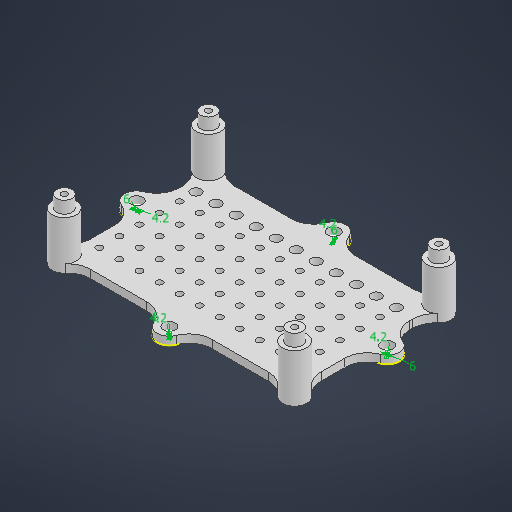
# Autodesk Inventor part: Bottom_Tip_Matrix
Saved by Autodesk Inventor 2025.1 (Build 291241000, 241)
## iProperties
Created: 2025-02-14
Part Number: Bottom_Tip_Matrix
Material: Generic
Document SubType Name: Modeling
Designer: m_kni
Density: 1 g/cm^3
Appearance: Default
Author: m_kni
## iProperties of the stored document Bottom_Tip_Matrix_3DPrint.ipt
Created: 2025-02-16
Part Number: Bottom_Tip_Matrix_3DPrint
Material: Generic
Document SubType Name: Modeling
Designer: m_kni
Density: 1 g/cm^3
Appearance: Default
Author: m_kni
Autodesk Inventor part; units mm, degrees
ref_plane "YZ Plane" through (0, 0, 0) normal (1, 0, 0) x (0, 1, 0)
ref_plane "XZ Plane" through (0, 0, 0) normal (0, 1, 0) x (-1, 0, 0)
ref_plane "XY Plane" through (0, 0, 0) normal (0, 0, 1) x (1, 0, 0)
sketch "Sketch1" plane through (0, 0, 0) normal (0, 1, 0) x (-1, 0, 0)
  line L0 (63.6935, -29.7828) -> (-51.3065, -29.7828)
  line L1 (-51.3065, -29.7828) -> (-51.3065, 42.2172)
  line L2 (-51.3065, 42.2172) -> (63.6935, 42.2172)
  line L3 (63.6935, -29.7828) -> (-51.3065, 42.2172) construction
  line L4 (-51.3065, -29.7828) -> (63.6935, 42.2172) construction
  circle A0 centre (-42.3065, 30.6406) radius 1.6
  circle A1 centre (-42.3065, 20.6406) radius 1.6
  circle A2 centre (-42.3065, 10.6406) radius 1.6
  circle A3 centre (-42.3065, 0.6406) radius 1.6
  circle A4 centre (-42.3065, -9.3594) radius 1.6
  circle A5 centre (-32.3065, 30.6406) radius 1.6
  circle A6 centre (-32.3065, 20.6406) radius 1.6
  circle A7 centre (-32.3065, 10.6406) radius 1.6
  circle A8 centre (-32.3065, 0.6406) radius 1.6
  circle A9 centre (-32.3065, -9.3594) radius 1.6
  circle A10 centre (-22.3065, 30.6406) radius 1.6
  circle A11 centre (-22.3065, 20.6406) radius 1.6
  circle A12 centre (-22.3065, 10.6406) radius 1.6
  circle A13 centre (-22.3065, 0.6406) radius 1.6
  circle A14 centre (-22.3065, -9.3594) radius 1.6
  circle A15 centre (-12.3065, 30.6406) radius 1.6
  circle A16 centre (-12.3065, 20.6406) radius 1.6
  circle A17 centre (-12.3065, 10.6406) radius 1.6
  circle A18 centre (-12.3065, 0.6406) radius 1.6
  circle A19 centre (-12.3065, -9.3594) radius 1.6
  circle A20 centre (-2.3065, 30.6406) radius 1.6
  circle A21 centre (-2.3065, 20.6406) radius 1.6
  circle A22 centre (-2.3065, 10.6406) radius 1.6
  circle A23 centre (-2.3065, 0.6406) radius 1.6
  circle A24 centre (-2.3065, -9.3594) radius 1.6
  circle A25 centre (7.6935, 30.6406) radius 1.6
  circle A26 centre (7.6935, 20.6406) radius 1.6
  circle A27 centre (7.6935, 10.6406) radius 1.6
  circle A28 centre (7.6935, 0.6406) radius 1.6
  circle A29 centre (7.6935, -9.3594) radius 1.6
  circle A30 centre (17.6935, 30.6406) radius 1.6
  circle A31 centre (17.6935, 20.6406) radius 1.6
  circle A32 centre (17.6935, 10.6406) radius 1.6
  circle A33 centre (17.6935, 0.6406) radius 1.6
  circle A34 centre (17.6935, -9.3594) radius 1.6
  circle A35 centre (27.6935, 30.6406) radius 1.6
  circle A36 centre (27.6935, 20.6406) radius 1.6
  circle A37 centre (27.6935, 10.6406) radius 1.6
  circle A38 centre (27.6935, 0.6406) radius 1.6
  circle A39 centre (27.6935, -9.3594) radius 1.6
  circle A40 centre (37.6935, 30.6406) radius 1.6
  circle A41 centre (37.6935, 20.6406) radius 1.6
  circle A42 centre (37.6935, 10.6406) radius 1.6
  circle A43 centre (37.6935, 0.6406) radius 1.6
  circle A44 centre (37.6935, -9.3594) radius 1.6
  circle A45 centre (47.6935, 30.6406) radius 1.6
  circle A46 centre (47.6935, 20.6406) radius 1.6
  circle A47 centre (47.6935, 10.6406) radius 1.6
  circle A48 centre (47.6935, 0.6406) radius 1.6
  circle A49 centre (47.6935, -9.3594) radius 1.6
  circle A50 centre (57.6935, 30.6406) radius 1.6
  circle A51 centre (57.6935, 20.6406) radius 1.6
  circle A52 centre (57.6935, 10.6406) radius 1.6
  circle A53 centre (57.6935, 0.6406) radius 1.6
  circle A54 centre (57.6935, -9.3594) radius 1.6
  line L5 (-51.3065, 42.2172) -> (63.6935, 42.2172)
  line L6 (63.6935, 42.2172) -> (63.6935, -29.7828)
  line L7 (63.6935, -29.7828) -> (-51.3065, -29.7828)
  line L8 (-51.3065, -29.7828) -> (-51.3065, 42.2172)
  circle A55 centre (-51.3065, 42.2172) radius 6
  circle A56 centre (-51.3065, -29.7828) radius 6
  circle A57 centre (63.6935, 42.2172) radius 6
  circle A58 centre (63.6935, -29.7828) radius 6
  circle A59 centre (57.6935, -17.5594) radius 2.5
  line L9 (57.6935, -9.3594) -> (57.6935, -17.5594) construction
  circle A60 centre (47.6935, -17.5594) radius 2.5
  circle A61 centre (37.6935, -17.5594) radius 2.5
  circle A62 centre (27.6935, -17.5594) radius 2.5
  circle A63 centre (17.6935, -17.5594) radius 2.5
  circle A64 centre (7.6935, -17.5594) radius 2.5
  circle A65 centre (-2.3065, -17.5594) radius 2.5
  circle A66 centre (-12.3065, -17.5594) radius 2.5
  circle A67 centre (-22.3065, -17.5594) radius 2.5
  circle A68 centre (-32.3065, -17.5594) radius 2.5
  circle A69 centre (-42.3065, -17.5594) radius 2.5
  point P0 (0, 0)
  point P1 (6.1935, 6.2172)
  point P2 (60.4545, 30.6406)
  point P3 (-45.5455, -35.3594)
  point P4 (63.6935, -23.7828)
  point P5 (63.6935, 36.2172)
  point P6 (57.6935, 42.2172)
  point P7 (-45.3065, 42.2172)
  point P8 (-51.3065, 36.2172)
  point P9 (-51.3065, -23.7828)
  point P10 (-45.3065, -29.7828)
  point P11 (57.6935, -29.7828)
  dimension "d4" = 115
  dimension "d5" = 72
  dimension "d6" = 3.2
  dimension "d9" = 10
  dimension "d10" = 10
  dimension "d13" = 12
  dimension "d14" = 12
  dimension "d15" = 12
  dimension "d16" = 12
  dimension "d58" = 6
  dimension "d59" = 8.2
  dimension "d60" = 5
  dimension "d63" = 10
  constraints: 70 centre point, 20 end point, 5 coincident, 4 horizontal, 3 parallel, 2 midpoint, 2 perpendicular, 2 vertical, 1 point on line, 128 other
  measures "d4" distance of L1.end L4.end
  measures "d5" distance of L1.start L1.end
  measures "d6" diameter of A0
  measures "d9" distance of A0.centre A1.centre
  measures "d10" distance of A0.centre A5.centre
  measures "d13" diameter of A55
  measures "d14" diameter of A56
  measures "d15" diameter of A57
  measures "d16" diameter of A58
  measures "d58" distance from line of L6 A50.centre
  measures "d59" distance of L9.start L9.end
  measures "d60" diameter of A59
  measures "d63" distance of L9.end A60.centre
extrude "Extrusion1" add sketch "Sketch1" along normal blind 4
sketch "Sketch2" plane through (0, 4, 0) normal (0, 1, 0) x (1, 0, 0)
  arc A0 (45.3065, -42.2172) -> (51.3065, -36.2172) centre (51.3065, -42.2172) ccw projected
  arc A1 (-63.6935, -36.2172) -> (-57.6935, -42.2172) centre (-63.6935, -42.2172) ccw projected
  arc A2 (-57.6935, 29.7828) -> (-63.6935, 23.7828) centre (-63.6935, 29.7828) ccw projected
  arc A3 (51.3065, 23.7828) -> (45.3065, 29.7828) centre (51.3065, 29.7828) ccw projected
  circle A4 centre (-63.6935, -42.2172) radius 6
  circle A5 centre (-63.6935, 29.7828) radius 6
  circle A6 centre (51.3065, -42.2172) radius 6
  circle A7 centre (51.3065, 29.7828) radius 6
  point P0 (0, 0)
  point P1 (51.3065, 23.7828)
  point P2 (45.3065, -42.2172)
  point P3 (-57.6935, 29.7828)
  constraints: 4 coincident, 3 centre point, 3 concentric, 3 other
extrude "Extrusion2" add sketch "Sketch2" along normal blind 20
sketch "Sketch3" plane through (51.3065, 24, 42.2172) normal (0, 1, 0) x (1, 0, 0)
  circle A0 centre (0, 0) radius 3.85
  arc A1 (0, 66) -> (-6, 72) centre (0, 72) ccw projected
  circle A2 centre (0, 72) radius 3.85
  arc A3 (-115, 6) -> (-109, 0) centre (-115, 0) ccw projected
  circle A4 centre (-115, 0) radius 3.85
  circle A5 centre (-115, 72) radius 3.85
  circle A6 centre (-115, 72) radius 6 projected
  point P0 (-51.3065, 42.2172)
  dimension "d21" = 7.7
  dimension "d22" = 7.7
  dimension "d23" = 7.7
  dimension "d24" = 7.7
  constraints: 4 centre point, 3 coincident
  measures "d21" diameter of A0
  measures "d22" diameter of A2
  measures "d23" diameter of A4
  measures "d24" diameter of A5
extrude "Extrusion3" add sketch "Sketch3" along normal blind 6 contours A0 | A2 | A4 | A5
sketch "Sketch4" plane through (-63.6935, 30, 42.2172) normal (0, 1, 0) x (1, 0, 0)
  circle A0 centre (0, 0) radius 3.85 projected
  circle A1 centre (0, 72) radius 3.85 projected
  circle A2 centre (115, 0) radius 3.85 projected
  circle A3 centre (115, 72) radius 3.85 projected
  circle A4 centre (0, 0) radius 1.5
  circle A5 centre (115, 0) radius 1.5
  circle A6 centre (0, 72) radius 1.5
  circle A7 centre (115, 72) radius 1.5
  point P0 (63.6935, 42.2172)
  dimension "d27" = 3
  dimension "d28" = 3
  dimension "d29" = 3
  dimension "d30" = 3
  constraints: 4 centre point, 4 coincident
  measures "d27" diameter of A4
  measures "d28" diameter of A5
  measures "d29" diameter of A6
  measures "d30" diameter of A7
extrude "Extrusion4" cut sketch "Sketch4" against normal blind 8 contours A4 | A5 | A6 | A7
sketch "Sketch5" plane through (0, 4, 0) normal (0, 1, 0) x (1, 0, 0)
  line L0 (-57.6935, -42.2172) -> (45.3065, -42.2172) projected
  line L1 (-6.1935, -42.2172) -> (-6.1935, -47.2172)
  circle A0 centre (-6.1935, -47.2172) radius 6
  line L2 (45.3065, 29.7828) -> (-57.6935, 29.7828) projected
  line L3 (-63.6935, 23.7828) -> (-63.6935, -36.2172) projected
  line L4 (51.3065, -36.2172) -> (51.3065, 23.7828) projected
  circle A1 centre (56.3065, -1.0083) radius 6
  circle A2 centre (-6.1935, 34.7828) radius 6
  circle A3 centre (-68.6935, -1.0083) radius 6
  line L5 (56.3065, -7.0083) -> (51.3065, -7.0083)
  line L6 (56.3065, 4.9917) -> (51.3065, 4.9917)
  line L7 (-68.6935, 4.9917) -> (-63.6935, 4.9917)
  line L8 (-68.6935, -7.0083) -> (-63.6935, -7.0083)
  line L9 (-12.1935, -47.2172) -> (-12.1935, -42.2172)
  line L10 (-0.1935, -47.2172) -> (-0.1935, -42.2172)
  line L11 (-12.1935, 34.7828) -> (-12.1935, 29.7828)
  line L12 (-0.1935, 34.7828) -> (-0.1935, 29.7828)
  line L13 (-12.1935, -42.2172) -> (-12.7108, -42.2172)
  circle A4 centre (42.3065, -10.6406) radius 1.6 projected
  circle A5 centre (42.3065, -0.6406) radius 1.6 projected
  circle A6 centre (32.3065, -10.6406) radius 1.6 projected
  circle A7 centre (32.3065, -30.6406) radius 1.6 projected
  circle A8 centre (32.3065, -10.6406) radius 1.6 projected
  circle A9 centre (32.3065, 9.3594) radius 1.6 projected
  circle A10 centre (32.3065, 9.3594) radius 1.6 projected
  circle A11 centre (32.3065, 9.3594) radius 1.6 projected
  circle A12 centre (32.3065, 9.3594) radius 1.6 projected
  circle A13 centre (32.3065, 19.3594) radius 1.6 projected
  circle A14 centre (42.3065, 9.3594) radius 1.6 projected
  arc A15 (45.3065, -42.2172) -> (51.3065, -36.2172) centre (51.3065, -42.2172) ccw projected
  arc A16 (51.3065, -36.2172) -> (45.3065, -42.2172) centre (51.3065, -42.2172) ccw projected
  arc A17 (45.3065, 29.7828) -> (51.3065, 23.7828) centre (51.3065, 29.7828) ccw projected
  circle A18 centre (2.3065, 19.3594) radius 1.6 projected
  circle A19 centre (2.3065, 19.3594) radius 1.6 projected
  circle A20 centre (51.3065, 29.7828) radius 3.85 projected
  circle A21 centre (51.3065, 29.7828) radius 1.5 projected
  circle A22 centre (51.3065, 29.7828) radius 1.5 projected
  circle A23 centre (51.3065, 29.7828) radius 1.5 projected
  circle A24 centre (51.3065, 29.7828) radius 3.85 projected
  circle A25 centre (51.3065, 29.7828) radius 1.5 projected
  circle A26 centre (51.3065, 29.7828) radius 1.5 projected
  circle A27 centre (51.3065, 29.7828) radius 1.5 projected
  circle A28 centre (2.3065, 29.3594) radius 1.6 projected
  circle A29 centre (2.3065, 29.3594) radius 1.6 projected
  circle A30 centre (2.3065, 29.3594) radius 1.6 projected
  circle A31 centre (2.3065, 29.3594) radius 1.6 projected
  circle A32 centre (12.3065, 29.3594) radius 1.6 projected
  circle A33 centre (12.3065, 29.3594) radius 1.6 projected
  circle A34 centre (12.3065, 9.3594) radius 1.6 projected
  circle A35 centre (12.3065, 9.3594) radius 1.6 projected
  circle A36 centre (12.3065, 9.3594) radius 1.6 projected
  circle A37 centre (12.3065, 9.3594) radius 1.6 projected
  circle A38 centre (12.3065, 19.3594) radius 1.6 projected
  circle A39 centre (12.3065, 19.3594) radius 1.6 projected
  circle A40 centre (12.3065, 19.3594) radius 1.6 projected
  circle A41 centre (12.3065, 29.3594) radius 1.6 projected
  circle A42 centre (12.3065, 29.3594) radius 1.6 projected
  circle A43 centre (2.3065, 9.3594) radius 1.6 projected
  circle A44 centre (2.3065, 9.3594) radius 1.6 projected
  circle A45 centre (2.3065, 19.3594) radius 1.6 projected
  circle A46 centre (2.3065, 19.3594) radius 1.6 projected
  circle A47 centre (2.3065, 9.3594) radius 1.6 projected
  circle A48 centre (12.3065, 19.3594) radius 1.6 projected
  circle A49 centre (22.3065, 29.3594) radius 1.6 projected
  arc A50 (51.3065, 23.7828) -> (45.3065, 29.7828) centre (51.3065, 29.7828) ccw projected
  circle A51 centre (22.3065, 9.3594) radius 1.6 projected
  circle A52 centre (-7.6935, -0.6406) radius 1.6 projected
  circle A53 centre (-7.6935, -0.6406) radius 1.6 projected
  circle A54 centre (-7.6935, -10.6406) radius 1.6 projected
  circle A55 centre (-17.6935, -10.6406) radius 1.6 projected
  circle A56 centre (-17.6935, -10.6406) radius 1.6 projected
  circle A57 centre (51.3065, -42.2172) radius 1.5 projected
  circle A58 centre (42.3065, 9.3594) radius 1.6 projected
  circle A59 centre (42.3065, 9.3594) radius 1.6 projected
  circle A60 centre (51.3065, -42.2172) radius 3.85 projected
  circle A61 centre (42.3065, 19.3594) radius 1.6 projected
  circle A62 centre (42.3065, 19.3594) radius 1.6 projected
  circle A63 centre (-7.6935, 9.3594) radius 1.6 projected
  circle A64 centre (-17.6935, 9.3594) radius 1.6 projected
  circle A65 centre (-17.6935, 9.3594) radius 1.6 projected
  circle A66 centre (-7.6935, 9.3594) radius 1.6 projected
  circle A67 centre (-7.6935, -20.6406) radius 1.6 projected
  circle A68 centre (-7.6935, -20.6406) radius 1.6 projected
  circle A69 centre (12.3065, -20.6406) radius 1.6 projected
  circle A70 centre (2.3065, -30.6406) radius 1.6 projected
  circle A71 centre (-7.6935, -30.6406) radius 1.6 projected
  circle A72 centre (-7.6935, -30.6406) radius 1.6 projected
  circle A73 centre (-17.6935, -20.6406) radius 1.6 projected
  circle A74 centre (-17.6935, -20.6406) radius 1.6 projected
  circle A75 centre (12.3065, -20.6406) radius 1.6 projected
  circle A76 centre (2.3065, -0.6406) radius 1.6 projected
  circle A77 centre (-17.6935, -30.6406) radius 1.6 projected
  circle A78 centre (-17.6935, -30.6406) radius 1.6 projected
  circle A79 centre (2.3065, -0.6406) radius 1.6 projected
  circle A80 centre (-7.6935, 19.3594) radius 1.6 projected
  circle A81 centre (-7.6935, 19.3594) radius 1.6 projected
  circle A82 centre (-7.6935, 29.3594) radius 1.6 projected
  circle A83 centre (-7.6935, 29.3594) radius 1.6 projected
  circle A84 centre (-17.6935, 19.3594) radius 1.6 projected
  circle A85 centre (-17.6935, 19.3594) radius 1.6 projected
  circle A86 centre (-7.6935, 19.3594) radius 1.6 projected
  circle A87 centre (-7.6935, 19.3594) radius 1.6 projected
  circle A88 centre (-7.6935, 29.3594) radius 1.6 projected
  circle A89 centre (-7.6935, 29.3594) radius 1.6 projected
  circle A90 centre (-17.6935, -0.6406) radius 1.6 projected
  circle A91 centre (-17.6935, -0.6406) radius 1.6 projected
  circle A92 centre (51.3065, -42.2172) radius 3.85 projected
  circle A93 centre (51.3065, -42.2172) radius 1.5 projected
  circle A94 centre (51.3065, -42.2172) radius 1.5 projected
  circle A95 centre (51.3065, -42.2172) radius 3.85 projected
  circle A96 centre (51.3065, -42.2172) radius 1.5 projected
  circle A97 centre (51.3065, -42.2172) radius 1.5 projected
  circle A98 centre (32.3065, -30.6406) radius 1.6 projected
  circle A99 centre (32.3065, -30.6406) radius 1.6 projected
  circle A100 centre (32.3065, -0.6406) radius 1.6 projected
  circle A101 centre (32.3065, -0.6406) radius 1.6 projected
  circle A102 centre (32.3065, -10.6406) radius 1.6 projected
  circle A103 centre (32.3065, -10.6406) radius 1.6 projected
  circle A104 centre (32.3065, -20.6406) radius 1.6 projected
  circle A105 centre (32.3065, -20.6406) radius 1.6 projected
  circle A106 centre (42.3065, -20.6406) radius 1.6 projected
  circle A107 centre (42.3065, -20.6406) radius 1.6 projected
  circle A108 centre (42.3065, -10.6406) radius 1.6 projected
  circle A109 centre (42.3065, -10.6406) radius 1.6 projected
  circle A110 centre (42.3065, -30.6406) radius 1.6 projected
  circle A111 centre (42.3065, -30.6406) radius 1.6 projected
  circle A112 centre (51.3065, -42.2172) radius 3.85 projected
  circle A113 centre (51.3065, -42.2172) radius 3.85 projected
  circle A114 centre (51.3065, -42.2172) radius 6 projected
  circle A115 centre (51.3065, -42.2172) radius 6 projected
  arc A116 (45.3065, -42.2172) -> (51.3065, -36.2172) centre (51.3065, -42.2172) ccw projected
  arc A117 (51.3065, -36.2172) -> (45.3065, -42.2172) centre (51.3065, -42.2172) ccw projected
  circle A118 centre (51.3065, -42.2172) radius 3.85 projected
  circle A119 centre (51.3065, -42.2172) radius 6 projected
  line L14 (51.3065, -36.2172) -> (51.3065, 23.7828) projected
  line L15 (51.3065, -36.2172) -> (51.3065, 23.7828) projected
  circle A120 centre (42.3065, -0.6406) radius 1.6 projected
  circle A121 centre (42.3065, -0.6406) radius 1.6 projected
  circle A122 centre (-27.6935, 19.3594) radius 1.6 projected
  circle A123 centre (-27.6935, 29.3594) radius 1.6 projected
  circle A124 centre (-27.6935, 29.3594) radius 1.6 projected
  circle A125 centre (-27.6935, 19.3594) radius 1.6 projected
  circle A126 centre (-47.6935, -20.6406) radius 1.6 projected
  circle A127 centre (-47.6935, -20.6406) radius 1.6 projected
  circle A128 centre (-47.6935, -30.6406) radius 1.6 projected
  circle A129 centre (-47.6935, -30.6406) radius 1.6 projected
  circle A130 centre (-37.6935, -20.6406) radius 1.6 projected
  circle A131 centre (-37.6935, -20.6406) radius 1.6 projected
  circle A132 centre (-27.6935, 9.3594) radius 1.6 projected
  circle A133 centre (-27.6935, 9.3594) radius 1.6 projected
  circle A134 centre (-37.6935, -0.6406) radius 1.6 projected
  circle A135 centre (-37.6935, -0.6406) radius 1.6 projected
  circle A136 centre (-27.6935, -30.6406) radius 1.6 projected
  circle A137 centre (-27.6935, -30.6406) radius 1.6 projected
  circle A138 centre (-27.6935, -10.6406) radius 1.6 projected
  circle A139 centre (-27.6935, -10.6406) radius 1.6 projected
  circle A140 centre (-27.6935, -0.6406) radius 1.6 projected
  circle A141 centre (-27.6935, -0.6406) radius 1.6 projected
  circle A142 centre (-37.6935, 9.3594) radius 1.6 projected
  circle A143 centre (-27.6935, -20.6406) radius 1.6 projected
  circle A144 centre (-27.6935, -20.6406) radius 1.6 projected
  circle A145 centre (-37.6935, -10.6406) radius 1.6 projected
  circle A146 centre (-37.6935, -10.6406) radius 1.6 projected
  circle A147 centre (-47.6935, -10.6406) radius 1.6 projected
  circle A148 centre (-37.6935, -30.6406) radius 1.6 projected
  circle A149 centre (-37.6935, -30.6406) radius 1.6 projected
  circle A150 centre (-37.6935, 9.3594) radius 1.6 projected
  circle A151 centre (-47.6935, -0.6406) radius 1.6 projected
  circle A152 centre (-47.6935, -0.6406) radius 1.6 projected
  circle A153 centre (-57.6935, 19.3594) radius 1.6 projected
  circle A154 centre (-57.6935, 19.3594) radius 1.6 projected
  circle A155 centre (-57.6935, 9.3594) radius 1.6 projected
  circle A156 centre (-57.6935, 9.3594) radius 1.6 projected
  circle A157 centre (-47.6935, 19.3594) radius 1.6 projected
  circle A158 centre (-47.6935, 19.3594) radius 1.6 projected
  circle A159 centre (-57.6935, -10.6406) radius 1.6 projected
  circle A160 centre (-37.6935, 19.3594) radius 1.6 projected
  circle A161 centre (-37.6935, 29.3594) radius 1.6 projected
  circle A162 centre (-37.6935, 29.3594) radius 1.6 projected
  circle A163 centre (-57.6935, -10.6406) radius 1.6 projected
  circle A164 centre (-37.6935, 19.3594) radius 1.6 projected
  circle A165 centre (-63.6935, -42.2172) radius 1.5 projected
  circle A166 centre (-63.6935, -42.2172) radius 1.5 projected
  circle A167 centre (-63.6935, -42.2172) radius 1.5 projected
  circle A168 centre (-63.6935, -42.2172) radius 1.5 projected
  circle A169 centre (-63.6935, -42.2172) radius 1.5 projected
  arc A170 (-57.6935, -42.2172) -> (-63.6935, -36.2172) centre (-63.6935, -42.2172) ccw projected
  arc A171 (-63.6935, -36.2172) -> (-57.6935, -42.2172) centre (-63.6935, -42.2172) ccw projected
  line L16 (-63.6935, 23.7828) -> (-63.6935, -36.2172) projected
  arc A172 (-63.6935, 23.7828) -> (-57.6935, 29.7828) centre (-63.6935, 29.7828) ccw projected
  arc A173 (-57.6935, 29.7828) -> (-63.6935, 23.7828) centre (-63.6935, 29.7828) ccw projected
  circle A174 centre (-63.6935, 29.7828) radius 3.85 projected
  circle A175 centre (-63.6935, 29.7828) radius 1.5 projected
  circle A176 centre (-63.6935, 29.7828) radius 1.5 projected
  circle A177 centre (-63.6935, 29.7828) radius 1.5 projected
  circle A178 centre (-63.6935, 29.7828) radius 3.85 projected
  circle A179 centre (-63.6935, 29.7828) radius 1.5 projected
  circle A180 centre (-63.6935, 29.7828) radius 1.5 projected
  circle A181 centre (-63.6935, 29.7828) radius 6 projected
  arc A182 (-57.6935, 29.7828) -> (-63.6935, 23.7828) centre (-63.6935, 29.7828) ccw projected
  arc A183 (-63.6935, 23.7828) -> (-57.6935, 29.7828) centre (-63.6935, 29.7828) ccw projected
  circle A184 centre (-57.6935, 19.3594) radius 1.6 projected
  circle A185 centre (-57.6935, 19.3594) radius 1.6 projected
  circle A186 centre (-57.6935, 9.3594) radius 1.6 projected
  circle A187 centre (-57.6935, 9.3594) radius 1.6 projected
  circle A188 centre (-47.6935, 19.3594) radius 1.6 projected
  circle A189 centre (-47.6935, 19.3594) radius 1.6 projected
  circle A190 centre (-17.6935, 9.3594) radius 1.6 projected
  circle A191 centre (-17.6935, 9.3594) radius 1.6 projected
  circle A192 centre (-37.6935, 9.3594) radius 1.6 projected
  circle A193 centre (-37.6935, 9.3594) radius 1.6 projected
  circle A194 centre (-47.6935, 9.3594) radius 1.6 projected
  circle A195 centre (-47.6935, 9.3594) radius 1.6 projected
  circle A196 centre (-37.6935, 19.3594) radius 1.6 projected
  circle A197 centre (-37.6935, 19.3594) radius 1.6 projected
  circle A198 centre (-63.6935, 29.7828) radius 3.85 projected
  circle A199 centre (-63.6935, 29.7828) radius 3.85 projected
  circle A200 centre (-63.6935, 29.7828) radius 3.85 projected
  circle A201 centre (-63.6935, 29.7828) radius 6 projected
  circle A202 centre (-57.6935, 29.3594) radius 1.6 projected
  circle A203 centre (-57.6935, 29.3594) radius 1.6 projected
  circle A204 centre (-27.6935, 19.3594) radius 1.6 projected
  circle A205 centre (-27.6935, 19.3594) radius 1.6 projected
  circle A206 centre (-47.6935, 29.3594) radius 1.6 projected
  circle A207 centre (-47.6935, 29.3594) radius 1.6 projected
  circle A208 centre (-37.6935, 29.3594) radius 1.6 projected
  circle A209 centre (-37.6935, 29.3594) radius 1.6 projected
  circle A210 centre (-17.6935, 19.3594) radius 1.6 projected
  circle A211 centre (-17.6935, 19.3594) radius 1.6 projected
  circle A212 centre (-27.6935, 29.3594) radius 1.6 projected
  circle A213 centre (-27.6935, 29.3594) radius 1.6 projected
  circle A214 centre (-17.6935, 29.3594) radius 1.6 projected
  circle A215 centre (-17.6935, 29.3594) radius 1.6 projected
  circle A216 centre (-27.6935, 9.3594) radius 1.6 projected
  circle A217 centre (-27.6935, 9.3594) radius 1.6 projected
  circle A218 centre (-63.6935, -42.2172) radius 3.85 projected
  circle A219 centre (-63.6935, -42.2172) radius 1.5 projected
  circle A220 centre (-63.6935, -42.2172) radius 3.85 projected
  circle A221 centre (-63.6935, -42.2172) radius 3.85 projected
  circle A222 centre (-63.6935, -42.2172) radius 6 projected
  arc A223 (-63.6935, -36.2172) -> (-57.6935, -42.2172) centre (-63.6935, -42.2172) ccw projected
  arc A224 (-57.6935, -42.2172) -> (-63.6935, -36.2172) centre (-63.6935, -42.2172) ccw projected
  line L17 (-63.6935, 23.7828) -> (-63.6935, -36.2172) projected
  line L18 (-63.6935, 23.7828) -> (-63.6935, -36.2172) projected
  circle A225 centre (-47.6935, -0.6406) radius 1.6 projected
  circle A226 centre (-47.6935, -0.6406) radius 1.6 projected
  circle A227 centre (-57.6935, -10.6406) radius 1.6 projected
  circle A228 centre (-57.6935, -10.6406) radius 1.6 projected
  circle A229 centre (-47.6935, -20.6406) radius 1.6 projected
  circle A230 centre (-47.6935, -20.6406) radius 1.6 projected
  circle A231 centre (-47.6935, -30.6406) radius 1.6 projected
  circle A232 centre (-47.6935, -30.6406) radius 1.6 projected
  circle A233 centre (-37.6935, -20.6406) radius 1.6 projected
  circle A234 centre (-37.6935, -20.6406) radius 1.6 projected
  circle A235 centre (-37.6935, -0.6406) radius 1.6 projected
  circle A236 centre (-37.6935, -0.6406) radius 1.6 projected
  circle A237 centre (-17.6935, -0.6406) radius 1.6 projected
  circle A238 centre (-17.6935, -0.6406) radius 1.6 projected
  circle A239 centre (-27.6935, -0.6406) radius 1.6 projected
  circle A240 centre (-27.6935, -0.6406) radius 1.6 projected
  circle A241 centre (-57.6935, -0.6406) radius 1.6 projected
  circle A242 centre (-57.6935, -0.6406) radius 1.6 projected
  circle A243 centre (-27.6935, -10.6406) radius 1.6 projected
  circle A244 centre (-27.6935, -10.6406) radius 1.6 projected
  circle A245 centre (-17.6935, -10.6406) radius 1.6 projected
  circle A246 centre (-17.6935, -10.6406) radius 1.6 projected
  circle A247 centre (-47.6935, -10.6406) radius 1.6 projected
  circle A248 centre (-47.6935, -10.6406) radius 1.6 projected
  circle A249 centre (-17.6935, -20.6406) radius 1.6 projected
  circle A250 centre (-17.6935, -20.6406) radius 1.6 projected
  circle A251 centre (-27.6935, -20.6406) radius 1.6 projected
  circle A252 centre (-27.6935, -20.6406) radius 1.6 projected
  circle A253 centre (-17.6935, -30.6406) radius 1.6 projected
  circle A254 centre (-17.6935, -30.6406) radius 1.6 projected
  circle A255 centre (-27.6935, -30.6406) radius 1.6 projected
  circle A256 centre (-27.6935, -30.6406) radius 1.6 projected
  circle A257 centre (-37.6935, -30.6406) radius 1.6 projected
  circle A258 centre (-37.6935, -30.6406) radius 1.6 projected
  circle A259 centre (-57.6935, -20.6406) radius 1.6 projected
  circle A260 centre (-57.6935, -20.6406) radius 1.6 projected
  circle A261 centre (-57.6935, -30.6406) radius 1.6 projected
  circle A262 centre (-57.6935, -30.6406) radius 1.6 projected
  circle A263 centre (-63.6935, -42.2172) radius 3.85 projected
  circle A264 centre (-63.6935, -42.2172) radius 3.85 projected
  circle A265 centre (-63.6935, -42.2172) radius 3.85 projected
  circle A266 centre (-63.6935, -42.2172) radius 6 projected
  circle A267 centre (-37.6935, -10.6406) radius 1.6 projected
  circle A268 centre (-37.6935, -10.6406) radius 1.6 projected
  circle A269 centre (-47.6935, -10.6406) radius 1.6 projected
  circle A270 centre (-47.6935, 29.3594) radius 1.6 projected
  circle A271 centre (-47.6935, 29.3594) radius 1.6 projected
  circle A272 centre (-47.6935, 9.3594) radius 1.6 projected
  circle A273 centre (-57.6935, 29.3594) radius 1.6 projected
  circle A274 centre (-57.6935, 29.3594) radius 1.6 projected
  circle A275 centre (-63.6935, 29.7828) radius 3.85 projected
  circle A276 centre (-63.6935, 29.7828) radius 6 projected
  circle A277 centre (-57.6935, -0.6406) radius 1.6 projected
  circle A278 centre (-57.6935, -0.6406) radius 1.6 projected
  circle A279 centre (-57.6935, -20.6406) radius 1.6 projected
  circle A280 centre (-57.6935, -20.6406) radius 1.6 projected
  circle A281 centre (-57.6935, -30.6406) radius 1.6 projected
  circle A282 centre (-57.6935, -30.6406) radius 1.6 projected
  circle A283 centre (-63.6935, -42.2172) radius 6 projected
  circle A284 centre (-47.6935, 9.3594) radius 1.6 projected
  circle A285 centre (22.3065, 29.3594) radius 1.6 projected
  circle A286 centre (42.3065, -0.6406) radius 1.6 projected
  circle A287 centre (22.3065, 9.3594) radius 1.6 projected
  circle A288 centre (22.3065, 9.3594) radius 1.6 projected
  circle A289 centre (22.3065, 9.3594) radius 1.6 projected
  circle A290 centre (32.3065, -0.6406) radius 1.6 projected
  circle A291 centre (32.3065, -0.6406) radius 1.6 projected
  circle A292 centre (22.3065, -0.6406) radius 1.6 projected
  circle A293 centre (42.3065, -10.6406) radius 1.6 projected
  circle A294 centre (22.3065, -0.6406) radius 1.6 projected
  circle A295 centre (12.3065, -0.6406) radius 1.6 projected
  circle A296 centre (12.3065, -0.6406) radius 1.6 projected
  circle A297 centre (12.3065, -10.6406) radius 1.6 projected
  circle A298 centre (12.3065, -10.6406) radius 1.6 projected
  line L19 (51.3065, -36.2172) -> (51.3065, 23.7828) projected
  circle A299 centre (-17.6935, 29.3594) radius 1.6 projected
  circle A300 centre (-17.6935, 29.3594) radius 1.6 projected
  circle A301 centre (51.3065, -42.2172) radius 1.5 projected
  circle A302 centre (22.3065, -30.6406) radius 1.6 projected
  circle A303 centre (22.3065, -30.6406) radius 1.6 projected
  circle A304 centre (12.3065, -30.6406) radius 1.6 projected
  line L20 (45.3065, 29.7828) -> (-57.6935, 29.7828) projected
  line L21 (45.3065, 29.7828) -> (-57.6935, 29.7828) projected
  line L22 (45.3065, 29.7828) -> (-57.6935, 29.7828) projected
  circle A305 centre (-63.6935, 29.7828) radius 1.5 projected
  line L23 (-57.6935, -42.2172) -> (45.3065, -42.2172) projected
  line L24 (-57.6935, -42.2172) -> (45.3065, -42.2172) projected
  line L25 (-57.6935, -42.2172) -> (45.3065, -42.2172) projected
  arc A306 (51.3065, -36.2172) -> (45.3065, -42.2172) centre (51.3065, -42.2172) ccw projected
  line L26 (51.3065, -36.2172) -> (51.3065, 23.7828) projected
  arc A307 (45.3065, 29.7828) -> (51.3065, 23.7828) centre (51.3065, 29.7828) ccw projected
  line L27 (45.3065, 29.7828) -> (-57.6935, 29.7828) projected
  arc A308 (-63.6935, 23.7828) -> (-57.6935, 29.7828) centre (-63.6935, 29.7828) ccw projected
  line L28 (-63.6935, 23.7828) -> (-63.6935, -36.2172) projected
  arc A309 (-57.6935, -42.2172) -> (-63.6935, -36.2172) centre (-63.6935, -42.2172) ccw projected
  line L29 (-57.6935, -42.2172) -> (45.3065, -42.2172) projected
  circle A310 centre (-47.6935, -0.6406) radius 1.6 projected
  circle A311 centre (-57.6935, 9.3594) radius 1.6 projected
  circle A312 centre (-57.6935, -10.6406) radius 1.6 projected
  circle A313 centre (-47.6935, -20.6406) radius 1.6 projected
  circle A314 centre (-47.6935, -30.6406) radius 1.6 projected
  circle A315 centre (-37.6935, -20.6406) radius 1.6 projected
  circle A316 centre (-27.6935, 9.3594) radius 1.6 projected
  circle A317 centre (-37.6935, -0.6406) radius 1.6 projected
  circle A318 centre (-27.6935, -30.6406) radius 1.6 projected
  circle A319 centre (-27.6935, -10.6406) radius 1.6 projected
  circle A320 centre (22.3065, -10.6406) radius 1.6 projected
  circle A321 centre (22.3065, -30.6406) radius 1.6 projected
  circle A322 centre (12.3065, -0.6406) radius 1.6 projected
  circle A323 centre (12.3065, -10.6406) radius 1.6 projected
  circle A324 centre (12.3065, 9.3594) radius 1.6 projected
  circle A325 centre (2.3065, -20.6406) radius 1.6 projected
  circle A326 centre (2.3065, -10.6406) radius 1.6 projected
  circle A327 centre (-17.6935, -30.6406) radius 1.6 projected
  circle A328 centre (32.3065, -30.6406) radius 1.6 projected
  circle A329 centre (42.3065, -20.6406) radius 1.6 projected
  circle A330 centre (2.3065, -0.6406) radius 1.6 projected
  circle A331 centre (-17.6935, 9.3594) radius 1.6 projected
  circle A332 centre (-7.6935, 9.3594) radius 1.6 projected
  circle A333 centre (12.3065, -30.6406) radius 1.6 projected
  circle A334 centre (42.3065, -10.6406) radius 1.6 projected
  circle A335 centre (22.3065, -0.6406) radius 1.6 projected
  circle A336 centre (42.3065, -0.6406) radius 1.6 projected
  circle A337 centre (32.3065, -0.6406) radius 1.6 projected
  circle A338 centre (42.3065, 9.3594) radius 1.6 projected
  circle A339 centre (32.3065, 9.3594) radius 1.6 projected
  circle A340 centre (-7.6935, -0.6406) radius 1.6 projected
  circle A341 centre (-17.6935, -10.6406) radius 1.6 projected
  circle A342 centre (32.3065, -20.6406) radius 1.6 projected
  circle A343 centre (-17.6935, -20.6406) radius 1.6 projected
  circle A344 centre (-17.6935, -0.6406) radius 1.6 projected
  circle A345 centre (-7.6935, -20.6406) radius 1.6 projected
  circle A346 centre (-7.6935, -30.6406) radius 1.6 projected
  circle A347 centre (-7.6935, -10.6406) radius 1.6 projected
  circle A348 centre (22.3065, 9.3594) radius 1.6 projected
  circle A349 centre (2.3065, -30.6406) radius 1.6 projected
  circle A350 centre (12.3065, -20.6406) radius 1.6 projected
  circle A351 centre (22.3065, -20.6406) radius 1.6 projected
  circle A352 centre (32.3065, -10.6406) radius 1.6 projected
  circle A353 centre (2.3065, 9.3594) radius 1.6 projected
  circle A354 centre (-27.6935, -20.6406) radius 1.6 projected
  circle A355 centre (-27.6935, -0.6406) radius 1.6 projected
  circle A356 centre (-37.6935, 9.3594) radius 1.6 projected
  circle A357 centre (-37.6935, -10.6406) radius 1.6 projected
  circle A358 centre (-37.6935, -30.6406) radius 1.6 projected
  circle A359 centre (-47.6935, -10.6406) radius 1.6 projected
  circle A360 centre (-57.6935, -20.6406) radius 1.6 projected
  circle A361 centre (-47.6935, 9.3594) radius 1.6 projected
  circle A362 centre (-57.6935, -0.6406) radius 1.6 projected
  circle A363 centre (-57.6935, -30.6406) radius 1.6 projected
  circle A364 centre (42.3065, -30.6406) radius 1.6 projected
  arc A365 (-63.6935, -36.2172) -> (-57.6935, -42.2172) centre (-63.6935, -42.2172) ccw projected
  line L30 (-63.6935, 23.7828) -> (-63.6935, -36.2172) projected
  arc A366 (-57.6935, 29.7828) -> (-63.6935, 23.7828) centre (-63.6935, 29.7828) ccw projected
  line L31 (45.3065, 29.7828) -> (-57.6935, 29.7828) projected
  arc A367 (51.3065, 23.7828) -> (45.3065, 29.7828) centre (51.3065, 29.7828) ccw projected
  line L32 (51.3065, -36.2172) -> (51.3065, 23.7828) projected
  arc A368 (45.3065, -42.2172) -> (51.3065, -36.2172) centre (51.3065, -42.2172) ccw projected
  line L33 (-57.6935, -42.2172) -> (45.3065, -42.2172) projected
  circle A369 centre (-47.6935, -0.6406) radius 1.6 projected
  circle A370 centre (-57.6935, 9.3594) radius 1.6 projected
  circle A371 centre (-57.6935, -10.6406) radius 1.6 projected
  circle A372 centre (-47.6935, -20.6406) radius 1.6 projected
  circle A373 centre (-47.6935, -30.6406) radius 1.6 projected
  circle A374 centre (-37.6935, -20.6406) radius 1.6 projected
  circle A375 centre (-27.6935, 9.3594) radius 1.6 projected
  circle A376 centre (-37.6935, -0.6406) radius 1.6 projected
  circle A377 centre (-27.6935, -30.6406) radius 1.6 projected
  circle A378 centre (-27.6935, -10.6406) radius 1.6 projected
  circle A379 centre (22.3065, -10.6406) radius 1.6 projected
  circle A380 centre (22.3065, -30.6406) radius 1.6 projected
  circle A381 centre (12.3065, -0.6406) radius 1.6 projected
  circle A382 centre (12.3065, -10.6406) radius 1.6 projected
  circle A383 centre (12.3065, 9.3594) radius 1.6 projected
  circle A384 centre (2.3065, -20.6406) radius 1.6 projected
  circle A385 centre (2.3065, -10.6406) radius 1.6 projected
  circle A386 centre (-17.6935, -30.6406) radius 1.6 projected
  circle A387 centre (32.3065, -30.6406) radius 1.6 projected
  circle A388 centre (42.3065, -20.6406) radius 1.6 projected
  circle A389 centre (2.3065, -0.6406) radius 1.6 projected
  circle A390 centre (-17.6935, 9.3594) radius 1.6 projected
  circle A391 centre (-7.6935, 9.3594) radius 1.6 projected
  circle A392 centre (12.3065, -30.6406) radius 1.6 projected
  circle A393 centre (42.3065, -10.6406) radius 1.6 projected
  circle A394 centre (22.3065, -0.6406) radius 1.6 projected
  circle A395 centre (42.3065, -0.6406) radius 1.6 projected
  circle A396 centre (32.3065, -0.6406) radius 1.6 projected
  circle A397 centre (42.3065, 9.3594) radius 1.6 projected
  circle A398 centre (32.3065, 9.3594) radius 1.6 projected
  circle A399 centre (-7.6935, -0.6406) radius 1.6 projected
  circle A400 centre (-17.6935, -10.6406) radius 1.6 projected
  circle A401 centre (32.3065, -20.6406) radius 1.6 projected
  circle A402 centre (-17.6935, -20.6406) radius 1.6 projected
  circle A403 centre (-17.6935, -0.6406) radius 1.6 projected
  circle A404 centre (-7.6935, -20.6406) radius 1.6 projected
  circle A405 centre (-7.6935, -30.6406) radius 1.6 projected
  circle A406 centre (-7.6935, -10.6406) radius 1.6 projected
  circle A407 centre (22.3065, 9.3594) radius 1.6 projected
  circle A408 centre (2.3065, -30.6406) radius 1.6 projected
  circle A409 centre (12.3065, -20.6406) radius 1.6 projected
  circle A410 centre (22.3065, -20.6406) radius 1.6 projected
  circle A411 centre (32.3065, -10.6406) radius 1.6 projected
  circle A412 centre (2.3065, 9.3594) radius 1.6 projected
  circle A413 centre (-27.6935, -20.6406) radius 1.6 projected
  circle A414 centre (-27.6935, -0.6406) radius 1.6 projected
  circle A415 centre (-37.6935, 9.3594) radius 1.6 projected
  circle A416 centre (-37.6935, -10.6406) radius 1.6 projected
  circle A417 centre (-37.6935, -30.6406) radius 1.6 projected
  circle A418 centre (-47.6935, -10.6406) radius 1.6 projected
  circle A419 centre (-57.6935, -20.6406) radius 1.6 projected
  circle A420 centre (-47.6935, 9.3594) radius 1.6 projected
  circle A421 centre (-57.6935, -0.6406) radius 1.6 projected
  circle A422 centre (-57.6935, -30.6406) radius 1.6 projected
  circle A423 centre (42.3065, -30.6406) radius 1.6 projected
  circle A424 centre (22.3065, -10.6406) radius 1.6 projected
  circle A425 centre (12.3065, -30.6406) radius 1.6 projected
  circle A426 centre (2.3065, -30.6406) radius 1.6 projected
  circle A427 centre (-7.6935, -10.6406) radius 1.6 projected
  circle A428 centre (2.3065, 9.3594) radius 1.6 projected
  circle A429 centre (22.3065, -10.6406) radius 1.6 projected
  circle A430 centre (2.3065, -20.6406) radius 1.6 projected
  circle A431 centre (2.3065, -20.6406) radius 1.6 projected
  circle A432 centre (22.3065, -10.6406) radius 1.6 projected
  circle A433 centre (22.3065, -10.6406) radius 1.6 projected
  circle A434 centre (22.3065, -30.6406) radius 1.6 projected
  circle A435 centre (22.3065, -30.6406) radius 1.6 projected
  circle A436 centre (22.3065, -0.6406) radius 1.6 projected
  circle A437 centre (22.3065, -0.6406) radius 1.6 projected
  circle A438 centre (22.3065, -20.6406) radius 1.6 projected
  circle A439 centre (22.3065, -20.6406) radius 1.6 projected
  circle A440 centre (12.3065, -0.6406) radius 1.6 projected
  circle A441 centre (12.3065, -0.6406) radius 1.6 projected
  circle A442 centre (12.3065, -10.6406) radius 1.6 projected
  circle A443 centre (12.3065, -10.6406) radius 1.6 projected
  circle A444 centre (12.3065, -20.6406) radius 1.6 projected
  circle A445 centre (12.3065, -20.6406) radius 1.6 projected
  circle A446 centre (12.3065, -30.6406) radius 1.6 projected
  circle A447 centre (12.3065, -30.6406) radius 1.6 projected
  circle A448 centre (2.3065, -10.6406) radius 1.6 projected
  circle A449 centre (2.3065, -20.6406) radius 1.6 projected
  circle A450 centre (2.3065, -20.6406) radius 1.6 projected
  circle A451 centre (2.3065, -10.6406) radius 1.6 projected
  circle A452 centre (2.3065, -10.6406) radius 1.6 projected
  circle A453 centre (2.3065, -0.6406) radius 1.6 projected
  circle A454 centre (2.3065, -0.6406) radius 1.6 projected
  circle A455 centre (-7.6935, 9.3594) radius 1.6 projected
  circle A456 centre (-7.6935, 9.3594) radius 1.6 projected
  circle A457 centre (-7.6935, -0.6406) radius 1.6 projected
  circle A458 centre (-7.6935, -0.6406) radius 1.6 projected
  circle A459 centre (2.3065, -30.6406) radius 1.6 projected
  circle A460 centre (2.3065, -30.6406) radius 1.6 projected
  circle A461 centre (-7.6935, -10.6406) radius 1.6 projected
  circle A462 centre (-7.6935, -10.6406) radius 1.6 projected
  circle A463 centre (-7.6935, -20.6406) radius 1.6 projected
  circle A464 centre (-7.6935, -20.6406) radius 1.6 projected
  circle A465 centre (-7.6935, -30.6406) radius 1.6 projected
  circle A466 centre (-7.6935, -30.6406) radius 1.6 projected
  circle A467 centre (2.3065, -10.6406) radius 1.6 projected
  circle A468 centre (42.3065, -20.6406) radius 1.6 projected
  circle A469 centre (42.3065, -20.6406) radius 1.6 projected
  circle A470 centre (32.3065, -20.6406) radius 1.6 projected
  circle A471 centre (32.3065, -20.6406) radius 1.6 projected
  circle A472 centre (32.3065, -30.6406) radius 1.6 projected
  circle A473 centre (22.3065, -20.6406) radius 1.6 projected
  circle A474 centre (42.3065, -30.6406) radius 1.6 projected
  circle A475 centre (42.3065, -30.6406) radius 1.6 projected
  circle A476 centre (22.3065, -20.6406) radius 1.6 projected
  circle A477 centre (22.3065, 19.3594) radius 1.6 projected
  circle A478 centre (32.3065, 19.3594) radius 1.6 projected
  circle A479 centre (32.3065, 29.3594) radius 1.6 projected
  circle A480 centre (42.3065, 19.3594) radius 1.6 projected
  circle A481 centre (42.3065, 19.3594) radius 1.6 projected
  circle A482 centre (32.3065, 29.3594) radius 1.6 projected
  circle A483 centre (22.3065, 19.3594) radius 1.6 projected
  circle A484 centre (42.3065, 29.3594) radius 1.6 projected
  circle A485 centre (42.3065, 29.3594) radius 1.6 projected
  circle A486 centre (32.3065, 19.3594) radius 1.6 projected
  circle A487 centre (32.3065, 19.3594) radius 1.6 projected
  circle A488 centre (42.3065, 29.3594) radius 1.6 projected
  circle A489 centre (42.3065, 29.3594) radius 1.6 projected
  circle A490 centre (32.3065, 29.3594) radius 1.6 projected
  circle A491 centre (32.3065, 29.3594) radius 1.6 projected
  circle A492 centre (22.3065, 29.3594) radius 1.6 projected
  circle A493 centre (22.3065, 29.3594) radius 1.6 projected
  circle A494 centre (51.3065, 29.7828) radius 3.85 projected
  circle A495 centre (51.3065, 29.7828) radius 3.85 projected
  circle A496 centre (51.3065, 29.7828) radius 3.85 projected
  circle A497 centre (51.3065, 29.7828) radius 6 projected
  circle A498 centre (51.3065, 29.7828) radius 6 projected
  arc A499 (51.3065, 23.7828) -> (45.3065, 29.7828) centre (51.3065, 29.7828) ccw projected
  arc A500 (45.3065, 29.7828) -> (51.3065, 23.7828) centre (51.3065, 29.7828) ccw projected
  circle A501 centre (51.3065, 29.7828) radius 3.85 projected
  circle A502 centre (51.3065, 29.7828) radius 6 projected
  circle A503 centre (22.3065, 19.3594) radius 1.6 projected
  circle A504 centre (22.3065, 19.3594) radius 1.6 projected
  circle A505 centre (42.3065, 9.3594) radius 1.6 projected
  point P0 (0, 0)
  point P1 (-63.6935, -6.2172)
  point P2 (51.3065, -6.2172)
  point P3 (-2.8769, -42.2172)
  point P4 (-58.6639, 26.5112)
  point P5 (-58.6639, 33.0544)
  dimension "d33" = 5
  dimension "d34" = 12
  dimension "d35" = 5
  dimension "d36" = 5
  dimension "d37" = 5
  dimension "d38" = 12
  dimension "d39" = 12
  dimension "d40" = 12
  constraints: 20 end point, 17 point on line, 8 point on circle, 4 centre point, 4 coincident, 4 tangent, 3 midpoint, 3 perpendicular, 1 parallel, 1 vertical, 6 other
  measures "d33" distance of L1.start L1.end
  measures "d34" diameter of A0
  measures "d35" distance from line of point (-6.194, 34.783) L2
  measures "d36" distance from line of L3 point (-68.694, -1.008)
  measures "d37" distance from line of point (56.306, -1.008) L4
  measures "d38" diameter of A1
  measures "d39" diameter of A2
  measures "d40" diameter of A3
extrude "Extrusion5" add sketch "Sketch5" against normal up to surface (4 mm away) contours L0 A0 L9 | L8 A3 L3 | L0 A0 | A3 L3 | L0 L10 A0 | A3 L7 L3 | L4 A1 L5 | L4 A1 | L4 L6 A1 | L11 A2 L2 | A2 L2 A82 | A82 L2 | L12 L2 A2 picked at (-6.1935, -49.5214) picked at (-67.7477, 0.754) picked at (55.0949, -1.5031) picked at (-5.5577, 37.3305)
sketch "Sketch6" plane through (0, 0, 0) normal (0, -1, 0) x (1, 0, 0)
  arc A0 (-68.6935, 7.0083) -> (-68.6935, -4.9917) centre (-68.6935, 1.0083) ccw projected
  circle A1 centre (-68.6935, 1.0083) radius 3
  arc A2 (-12.1935, -34.7828) -> (-0.1935, -34.7828) centre (-6.1935, -34.7828) ccw projected
  circle A3 centre (-6.1935, -34.7828) radius 3
  arc A4 (56.3065, -4.9917) -> (56.3065, 7.0083) centre (56.3065, 1.0083) ccw projected
  circle A5 centre (56.3065, 1.0083) radius 3
  arc A6 (-0.1935, 47.2172) -> (-12.1935, 47.2172) centre (-6.1935, 47.2172) ccw projected
  circle A7 centre (-6.1935, 47.2172) radius 3
  circle A8 centre (-6.1935, 47.2172) radius 2.1
  circle A9 centre (56.3065, 1.0083) radius 2.1
  circle A10 centre (-6.1935, -34.7828) radius 2.1
  circle A11 centre (-68.6935, 1.0083) radius 2.1
  point P0 (0, 0)
  dimension "d43" = 6
  dimension "d44" = 6
  dimension "d45" = 6
  dimension "d46" = 6
  dimension "d47" = 4.2
  dimension "d48" = 4.2
  dimension "d49" = 4.2
  dimension "d50" = 4.2
  constraints: 8 centre point, 8 coincident
  measures "d43" diameter of A1
  measures "d44" diameter of A3
  measures "d45" diameter of A5
  measures "d46" diameter of A7
  measures "d47" diameter of A8
  measures "d48" diameter of A9
  measures "d49" diameter of A10
  measures "d50" diameter of A11
extrude "Extrusion6" cut sketch "Sketch6" against normal blind 10 contours A1 | A3 | A5 | A7 | A8 | A9 | A10 | A11
fillet "Fillet1" radius 11.525 16 edges at (-57.6935, 2, 42.2172) (-0.1935, 2, 42.2172) (45.3065, 2, 42.2172) (-12.1935, 2, 42.2172) (-63.6935, 2, 36.2172) (-63.6935, 2, 7.0083) (-63.6935, 2, -4.9917) (-63.6935, 2, -23.7828) (-57.6935, 2, -29.7828) (-12.1935, 2, -29.7828) (-0.1935, 2, -29.7828) (45.3065, 2, -29.7828) (51.3065, 2, -23.7828) (51.3065, 2, -4.9917) (51.3065, 2, 7.0083) (51.3065, 2, 36.2172)
equation "\"d21\" = d23"
equation "\"d22\" = d23"
equation "\"d24\" = d23"
body "Solid1"
